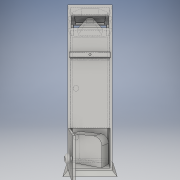
# Autodesk Inventor part: hologram display version 2
Saved by Autodesk Inventor 2016 (Build 200138000, 138)
## iProperties
Created: 2017-10-03
Part Number: hologram display version 2
Material: Generic
Document SubType Name: Modeling
Designer: student
Density: 1 g/cm^3
Appearance: Default
Author: student
Autodesk Inventor part; units mm, degrees
ref_plane "YZ Plane" through (0, 0, 0) normal (1, 0, 0) x (0, 1, 0)
ref_plane "XZ Plane" through (0, 0, 0) normal (0, 1, 0) x (-1, 0, 0)
sketch "Sketch1" plane through (0, 0, 0) normal (0, 0, 1) x (1, 0, 0)
  line L0 (-254, -861.9632) -> (254, -861.9632)
  line L1 (254, -861.9632) -> (254, 763.6368)
  line L2 (254, 763.6368) -> (-254, 763.6368)
  line L3 (-254, 763.6368) -> (-254, -861.9632)
  line L4 (-254, 763.6368) -> (254, 763.6368)
  line L5 (228.6, 763.6368) -> (228.6, -861.9632)
  line L6 (-228.6, 763.6368) -> (-228.6, -861.9632)
  line L7 (-228.6, -836.5632) -> (228.6, -836.5632)
  line L8 (-228.6, 738.2368) -> (228.6, 738.2368)
  line L9 (-254, -861.9632) -> (-304.8, -861.9632)
  line L10 (304.8, -861.9632) -> (304.8, -912.7632)
  line L11 (304.8, -912.7632) -> (-304.8, -912.7632)
  line L12 (-304.8, -912.7632) -> (-304.8, -861.9632)
  line L13 (254, -861.9632) -> (304.8, -861.9632)
  point P0 (0, 0)
  point P1 (0, 0)
  point P2 (0, 738.2368)
  dimension "d0" = 1625.6
  dimension "d1" = 508
  dimension "d3" = 25.4
  dimension "d4" = 25.4
  dimension "d5" = 25.4
  dimension "d6" = 25.4
  dimension "d7" = 50.8
  dimension "d8" = 50.8
  dimension "d19" = 50.8
  constraints: 28 end point, 8 point on line, 5 perpendicular, 4 horizontal, 3 parallel, 1 midpoint, 1 vertical alignment
  measures "d0" distance of L0.end L1.end
  measures "d1" distance of L0.start L0.end
  measures "d3" distance between parallel lines of L1 L5
  measures "d4" distance between parallel lines of L3 L6
  measures "d5" distance between parallel lines of L0 L7
  measures "d6" distance between parallel lines of L8 L2
  measures "d7" distance of L0.start L9.end
  measures "d8" distance of L10.start L10.end
  measures "d19" distance of L0.end L10.start
extrude "Extrusion1" add sketch "Sketch1" along normal blind 406.4 contours L3 L2 L6 L0 | L0 L13 L10 L11 L12 L9 | L6 L7 L5 L0 | L5 L2 L1 L0 | L2 L5 L8 L6
sketch "Sketch2" plane through (0, 0, 406.4) normal (0, 0, 1) x (1, 0, 0)
  line L0 (-304.8, -861.9632) -> (-304.8, -912.7632) projected
  line L1 (-304.8, -912.7632) -> (304.8, -912.7632) projected
  line L2 (-304.8, -861.9632) -> (304.8, -861.9632)
  line L3 (304.8, -861.9632) -> (304.8, -912.7632)
  line L4 (304.8, -912.7632) -> (-304.8, -912.7632)
  line L5 (-304.8, -912.7632) -> (-304.8, -861.9632)
  point P0 (0, 0)
  constraints: 8 end point, 2 parallel, 1 horizontal, 1 perpendicular
extrude "Extrusion2" add sketch "Sketch2" along normal blind 50.8
sketch "Sketch3" plane through (0, 0, 0) normal (0, 0, -1) x (-1, 0, 0)
  line L0 (-304.8, -912.7632) -> (-304.8, -861.9632) projected
  line L1 (304.8, -912.7632) -> (-304.8, -912.7632) projected
  line L2 (-304.8, -861.9632) -> (304.8, -861.9632)
  line L3 (304.8, -861.9632) -> (304.8, -912.7632)
  line L4 (304.8, -912.7632) -> (-304.8, -912.7632)
  line L5 (-304.8, -912.7632) -> (-304.8, -861.9632)
  point P0 (0, 0)
  constraints: 8 end point, 2 parallel, 1 horizontal, 1 perpendicular
extrude "Extrusion3" add sketch "Sketch3" along normal blind 50.8
sketch "Sketch4" plane through (228.6, -836.5632, 0) normal (-1, 0, 0) x (0, 0, 1)
  line L0 (0, 1574.8) -> (406.4, 1574.8) projected
  line L1 (0, 0) -> (25.4, 0)
  line L2 (25.4, 0) -> (25.4, 1574.8)
  line L3 (25.4, 1574.8) -> (0, 1574.8)
  line L4 (0, 1574.8) -> (0, 0)
  point P0 (0, 836.5632)
  dimension "d26" = 25.4
  constraints: 8 end point, 2 parallel, 1 horizontal, 1 perpendicular, 1 point on line
  measures "d26" distance between parallel lines of L4 L2
extrude "Extrusion4" add sketch "Sketch4" along normal blind 457.2
chamfer "Chamfer1" distance 50.8 angle 45 4 edges at (304.8, -861.9632, 203.2) (0, -861.9632, 457.2) (-304.8, -861.9632, 203.2) (0, -861.9632, -50.8)
sketch "Sketch5" plane through (-254, 763.6368, 0) normal (0, 1, 0) x (1, 0, 0)
  line L0 (403.225, -53.975) -> (403.225, -352.425)
  line L1 (403.225, -352.425) -> (104.775, -352.425)
  line L2 (104.775, -352.425) -> (104.775, -53.975)
  line L3 (104.775, -53.975) -> (403.225, -53.975)
  line L4 (508, 0) -> (0, 0) projected
  line L5 (508, 0) -> (508, -406.4) projected
  point P0 (254, 0)
  point P1 (254, -203.2)
  point P2 (254, 0)
  point P3 (508, -203.2)
  dimension "d32" = 298.45
  constraints: 8 end point, 2 midpoint, 1 horizontal alignment, 1 vertical alignment, 9 other
  measures "d32" distance of L0.start L0.end
ref_plane "Work Plane1" through (-254, 928.7368, 0) normal (0, 1, 0) x (1, 0, 0)
sketch "Sketch6" plane through (-254, 928.7368, 0) normal (0, 1, 0) x (1, 0, 0)
  line L0 (285.75, -171.45) -> (285.75, -234.95)
  line L1 (285.75, -234.95) -> (222.25, -234.95)
  line L2 (222.25, -234.95) -> (222.25, -171.45)
  line L3 (222.25, -171.45) -> (285.75, -171.45)
  line L4 (508, 0) -> (0, 0) projected
  line L5 (508, 0) -> (508, -406.4) projected
  point P0 (254, 0)
  point P1 (254, -203.2)
  point P2 (254, 0)
  point P3 (508, -203.2)
  dimension "d34" = 63.5
  constraints: 8 end point, 2 midpoint, 1 horizontal alignment, 1 parallel, 1 vertical alignment, 9 other
  measures "d34" distance of L0.start L0.end
loft "Loft1" add profiles "Sketch6", "Sketch5"
sketch "Sketch7" plane through (-31.75, 928.7368, 171.45) normal (0, 1, 0) x (1, 0, 0)
  line L0 (-173.99, 137.16) -> (237.49, 137.16)
  line L1 (237.49, 137.16) -> (237.49, -200.66)
  line L2 (237.49, -200.66) -> (-173.99, -200.66)
  line L3 (-173.99, -200.66) -> (-173.99, 137.16)
  line L4 (-173.99, 137.16) -> (237.49, -200.66) construction
  line L5 (237.49, 137.16) -> (-173.99, -200.66) construction
  line L6 (285.75, 171.45) -> (285.75, -234.95) projected
  point P0 (31.75, 171.45)
  point P1 (31.75, -31.75)
  point P2 (31.75, 137.16)
  point P3 (31.75, -31.75)
  point P4 (31.75, -31.75)
  point P5 (237.49, -31.75)
  point P6 (285.75, -31.75)
  dimension "d39" = 337.82
  dimension "d40" = 411.48
  constraints: 12 end point, 7 midpoint, 2 horizontal alignment, 2 parallel, 2 vertical alignment, 1 horizontal, 1 perpendicular
  measures "d39" distance of L0.end L1.end
  measures "d40" distance of L0.start L0.end
extrude "Extrusion5" add sketch "Sketch7" along normal blind 65.024
sketch "Sketch8" plane through (-205.74, 928.7368, 372.11) normal (0, 0, 1) x (1, 0, 0)
  line L0 (102.87, 65.024) -> (308.61, 65.024)
  line L1 (308.61, 65.024) -> (411.48, 23.876)
  line L2 (102.87, 65.024) -> (0, 23.876)
  line L3 (0, 23.876) -> (0, 65.024)
  line L4 (411.48, 65.024) -> (0, 65.024) projected
  line L5 (0, 65.024) -> (102.87, 65.024)
  line L6 (308.61, 65.024) -> (411.48, 65.024)
  line L7 (411.48, 65.024) -> (411.48, 23.876)
  point P0 (205.74, -928.7368)
  point P1 (205.74, 65.024)
  point P2 (205.74, 0)
  point P3 (411.48, 0)
  dimension "d49" = 205.74
  dimension "d50" = 23.876
  constraints: 14 end point, 3 perpendicular, 1 horizontal, 1 midpoint, 1 vertical alignment
  measures "d49" distance of L0.start L0.end
  measures "d50" distance of point (411.48, 0) L1.end
extrude "Extrusion6" cut sketch "Sketch8" against normal blind 649.351
sketch "Sketch9" plane through (-254, 763.6368, 0) normal (0, 1, 0) x (1, 0, 0)
  line L0 (508, 0) -> (0, 0) projected
  line L1 (38.1, 0) -> (38.1, -38.1)
  line L2 (38.1, -38.1) -> (0, -38.1)
  line L3 (0, -38.1) -> (0, 0)
  line L4 (0, 0) -> (38.1, 0)
  line L5 (508, 0) -> (508, -406.4) projected
  line L6 (508, 0) -> (508, -38.1)
  line L7 (508, -38.1) -> (469.9, -38.1)
  line L8 (469.9, -38.1) -> (469.9, 0)
  line L9 (469.9, 0) -> (508, 0)
  line L10 (0, 0) -> (0, -406.4) projected
  line L11 (0, -406.4) -> (0, -368.3)
  line L12 (0, -368.3) -> (38.1, -368.3)
  line L13 (38.1, -368.3) -> (38.1, -406.4)
  line L14 (38.1, -406.4) -> (0, -406.4)
  line L15 (508, -406.4) -> (469.9, -406.4)
  line L16 (469.9, -406.4) -> (469.9, -368.3)
  line L17 (469.9, -368.3) -> (508, -368.3)
  line L18 (508, -368.3) -> (508, -406.4)
  point P0 (254, 0)
  point P1 (19.05, -19.05)
  point P2 (19.05, 0)
  point P3 (0, -19.05)
  point P4 (488.95, -19.05)
  point P5 (488.95, 0)
  point P6 (19.05, -387.35)
  point P7 (19.05, -406.4)
  point P8 (488.95, -387.35)
  dimension "d53" = 38.1
  dimension "d54" = 38.1
  dimension "d55" = 38.1
  dimension "d56" = 38.1
  constraints: 32 end point, 4 midpoint, 3 horizontal alignment, 1 point on line, 1 vertical, 1 vertical alignment, 36 other
  measures "d53" distance of L1.start L1.end
  measures "d54" distance of L6.end L7.end
  measures "d55" distance of L12.end L13.end
  measures "d56" distance of L16.end L17.end
extrude "Extrusion7" add sketch "Sketch9" along normal blind 139.7
sketch "Sketch10" plane through (-254, 903.3368, 0) normal (0, 1, 0) x (1, 0, 0)
  line L0 (469.9, -406.4) -> (508, -406.4) projected
  line L1 (0, 0) -> (508, 0)
  line L2 (508, 0) -> (508, -406.4)
  line L3 (508, -406.4) -> (0, -406.4)
  line L4 (0, -406.4) -> (0, 0)
  line L5 (69.85, -31.75) -> (438.15, -31.75)
  line L6 (438.15, -31.75) -> (438.15, -374.65)
  line L7 (438.15, -374.65) -> (69.85, -374.65)
  line L8 (69.85, -374.65) -> (69.85, -31.75)
  line L9 (469.9, -368.3) -> (469.9, -406.4) projected
  line L10 (38.1, -406.4) -> (38.1, -368.3) projected
  line L11 (38.1, -38.1) -> (38.1, 0) projected
  line L12 (469.9, 0) -> (469.9, -38.1) projected
  point P0 (254, 0)
  dimension "d59" = 31.75
  dimension "d60" = 31.75
  dimension "d61" = 31.75
  dimension "d62" = 31.75
  dimension "d63" = 31.75
  dimension "d64" = 31.75
  constraints: 16 end point, 4 parallel, 2 horizontal, 2 perpendicular
  measures "d59" distance from line of L9 L6.end
  measures "d60" distance between parallel lines of L3 L7
  measures "d61" distance between parallel lines of L10 L8
  measures "d62" distance between parallel lines of L11 L8
  measures "d63" distance between parallel lines of L12 L6
  measures "d64" distance between parallel lines of L1 L5
extrude "Extrusion8" add sketch "Sketch10" along normal blind 25.4
sketch "Sketch11" plane through (-228.6, -836.5632, 406.4) normal (1, 0, 0) x (0, 0, -1)
  line L0 (0, 0) -> (0, 1574.8) projected
  line L1 (0, 1574.8) -> (25.4, 1574.8)
  line L2 (25.4, 1574.8) -> (25.4, 457.2)
  line L3 (25.4, 457.2) -> (0, 457.2)
  line L4 (0, 457.2) -> (0, 1574.8)
  line L5 (381, 0) -> (0, 0) projected
  point P0 (406.4, 836.5632)
  dimension "d67" = 25.4
  dimension "d68" = 457.2
  constraints: 8 end point, 2 parallel, 1 horizontal, 1 perpendicular
  measures "d67" distance between parallel lines of L0 L2
  measures "d68" distance between parallel lines of L5 L3
extrude "Extrusion9" add sketch "Sketch11" along normal blind 457.2
sketch "Sketch12" plane through (-254, 928.7368, 0) normal (0, 1, 0) x (1, 0, 0)
  line L0 (0, 0) -> (508, 0)
  line L1 (508, 0) -> (508, -406.4)
  line L2 (508, -406.4) -> (0, -406.4)
  line L3 (0, -406.4) -> (0, 0)
  line L4 (25.4, -25.4) -> (482.6, -25.4)
  line L5 (482.6, -25.4) -> (482.6, -381)
  line L6 (482.6, -381) -> (25.4, -381)
  line L7 (25.4, -381) -> (25.4, -25.4)
  line L8 (304.8, 0) -> (304.8, -25.4)
  line L9 (304.8, -25.4) -> (203.2, -25.4)
  line L10 (203.2, -25.4) -> (203.2, 0)
  point P0 (254, 0)
  dimension "d71" = 25.4
  dimension "d72" = 25.4
  dimension "d73" = 25.4
  dimension "d74" = 25.4
  constraints: 22 end point, 5 parallel, 3 point on line, 2 horizontal, 2 perpendicular
  measures "d71" distance between parallel lines of L0 L4
  measures "d72" distance between parallel lines of L3 L7
  measures "d73" distance between parallel lines of L1 L5
  measures "d74" distance between parallel lines of L2 L6
extrude "Extrusion10" add sketch "Sketch12" along normal blind 71.12 contours L0 L10 L4 L7 L6 L5 L8 L1 L2 L3
sketch "Sketch13" plane through (0, 0, 406.4) normal (0, 0, 1) x (1, 0, 0)
  line L0 (-254, 999.8568) -> (254, 999.8568) projected
  line L1 (-254, 999.8568) -> (254, 999.8568)
  line L2 (254, 999.8568) -> (254, 1025.2568)
  line L3 (254, 1025.2568) -> (-254, 1025.2568)
  line L4 (-254, 1025.2568) -> (-254, 999.8568)
  point P0 (0, 0)
  dimension "d78" = 25.4
  constraints: 8 end point, 2 parallel, 1 horizontal, 1 perpendicular
  measures "d78" distance of L1.end L2.end
extrude "Extrusion11" add sketch "Sketch13" against normal blind 406.4
sketch "Sketch14" plane through (-228.6, -836.5632, 406.4) normal (0, 1, 0) x (1, 0, 0)
  line L0 (3.5018, 227.1968) -> (364.1271, 13.6687)
  line L1 (364.1271, 13.6687) -> (451.4795, 161.1972)
  line L2 (451.4795, 161.1972) -> (90.8542, 374.7253)
  line L3 (90.8542, 374.7253) -> (3.5018, 227.1968)
  point P0 (228.6, 406.4)
  point P1 (234.9388, 199.449)
  dimension "d81" = 171.45
  dimension "d82" = 419.1
  constraints: 8 end point, 2 parallel, 1 perpendicular
  measures "d81" distance of L0.end L1.end
  measures "d82" distance of L0.start L0.end
extrude "Extrusion12" add sketch "Sketch14" along normal blind 355.6
fillet "Fillet1" radius 104.775 1 edges at (179.2033, -480.9632, 318.9671)
sketch "Sketch16" plane through (0, 0, 0) normal (0, 0, -1) x (-1, 0, 0)
  circle A0 centre (182.88, -557.1632) radius 38.1
  line L0 (-254, -861.9632) -> (254, -861.9632) projected
  line L1 (254, -861.9632) -> (254, 1025.2568) projected
  circle A1 centre (182.88, 77.8368) radius 38.1
  point P0 (0, 0)
  dimension "d95" = 304.8
  dimension "d96" = 76.2
  dimension "d99" = 71.12
  dimension "d100" = 939.8
  dimension "d136" = 71.12
  constraints: 2 centre point
  measures "d95" distance from line of L0 A0.centre
  measures "d96" diameter of A0
  measures "d99" distance from line of L1 A0.centre
  measures "d100" distance from line of L0 A1.centre
  measures "d136" distance from line of L1 A1.centre
extrude "Extrusion13" cut sketch "Sketch16" against normal blind 41.275
sketch "Sketch17" plane through (0, 0, 406.4) normal (0, 0, 1) x (1, 0, 0)
  line L0 (-254, 763.6368) -> (-215.9, 763.6368) projected
  line L1 (-228.6, 484.2368) -> (228.6, 484.2368)
  line L2 (228.6, 484.2368) -> (228.6, 420.7368)
  line L3 (228.6, -379.3632) -> (228.6, 738.2368) projected
  line L4 (228.6, 420.7368) -> (-228.6, 420.7368)
  line L5 (-228.6, 420.7368) -> (-228.6, 484.2368)
  line L6 (215.9, 763.6368) -> (-215.9, 763.6368) projected
  point P0 (0, 0)
  point P1 (0, 484.2368)
  point P2 (0, 763.6368)
  dimension "d104" = 63.5
  dimension "d113" = 457.2
  dimension "d114" = 279.4
  constraints: 8 end point, 2 midpoint, 2 perpendicular, 1 collinear, 1 horizontal, 1 vertical alignment
  measures "d104" distance of L4.end L1.start
  measures "d113" distance of L2.end L4.end
  measures "d114" distance between parallel lines of L6 L1
extrude "Extrusion14" cut sketch "Sketch17" against normal blind 98.425
sketch "Sketch18" plane through (0, 0, 406.4) normal (0, 0, 1) x (1, 0, 0)
  line L0 (228.6, 484.2368) -> (228.6, 420.7368) projected
  line L1 (-228.6, 420.7368) -> (228.6, 420.7368)
  line L2 (228.6, 420.7368) -> (228.6, 433.4368)
  line L3 (228.6, 433.4368) -> (-228.6, 433.4368)
  line L4 (-228.6, 433.4368) -> (-228.6, 420.7368)
  point P0 (0, 0)
  dimension "d107" = 12.7
  constraints: 8 end point, 2 parallel, 1 horizontal, 1 perpendicular, 1 point on line
  measures "d107" distance of L3.end L1.start
extrude "Extrusion15" add sketch "Sketch18" against normal blind 266.7 and the other way blind 76.2
sketch "Sketch19" plane through (-228.6, 433.4368, 406.4) normal (0, 1, 0) x (1, 0, 0)
  line L0 (0, 0) -> (0, -76.2) projected
  line L1 (0, 266.7) -> (0, 254)
  line L2 (457.2, 266.7) -> (0, 266.7)
  line L3 (0, 266.7) -> (0, 254)
  line L4 (0, 254) -> (457.2, 254)
  line L5 (457.2, 254) -> (457.2, 266.7)
  point P0 (228.6, 406.4)
  point P1 (0, 25.4)
  point P2 (0, 368.3)
  dimension "d115" = 12.7
  constraints: 10 end point, 2 parallel, 1 horizontal, 1 perpendicular, 1 point on line
  measures "d115" distance of L4.end L2.start
extrude "Extrusion16" add sketch "Sketch19" along normal blind 12.7
sketch "Sketch20" plane through (-228.6, -836.5632, 406.4) normal (0, 1, 0) x (1, 0, 0)
  line L0 (457.2, 0) -> (0, 0) projected
  line L1 (0, 0) -> (89.0436, -448.4452)
  line L2 (89.0436, -448.4452) -> (64.13, -453.392)
  line L3 (64.13, -453.392) -> (-24.9136, -4.9469)
  line L4 (-24.9136, -4.9469) -> (0, 0)
  point P0 (228.6, 406.4)
  dimension "d116" = 457.2
  dimension "d117" = 25.4
  constraints: 8 end point, 2 parallel, 1 perpendicular
  measures "d116" distance of L0.end L1.end
  measures "d117" distance of L1.end L2.end
extrude "Extrusion17" add sketch "Sketch20" along normal blind 457.2
sketch "Sketch21" plane through (-164.47, -836.5632, 859.792) normal (-0.9808512, 0, 0.1947586) x (0.1947586, 0, 0.9808512)
  circle A0 centre (-50.8, 228.6) radius 19.05
  line L0 (0, 0) -> (0, 457.2) projected
  point P0 (-811.2961, 836.5632)
  point P1 (0, 228.6)
  dimension "d120" = 38.1
  dimension "d135" = 50.8
  constraints: 1 centre point, 1 horizontal alignment, 1 midpoint
  measures "d120" diameter of A0
  measures "d135" distance of point (0, 228.6) A0.centre
extrude "Extrusion18" add sketch "Sketch21" along normal blind 19.05
sketch "Sketch22" plane through (-193.0489, -607.9632, 813.6749) normal (-0.9808512, 0, 0.1947586) x (0.1947586, 0, 0.9808512)
  circle A0 centre (0, 0) radius 19.05 projected
  circle A1 centre (0, 0) radius 50.8
  point P0 (-760.4961, 607.9632)
  dimension "d123" = 101.6
  constraints: 1 centre point, 1 coincident
  measures "d123" diameter of A1
extrude "Extrusion19" add sketch "Sketch22" along normal blind 50.8 contours A0 | A1
fillet "Fillet2" radius 25.4 2 edges at (-202.9427, -607.9632, 763.8477) (-252.7699, -607.9632, 773.7414)
sketch "Sketch23" plane through (-228.6, 433.4368, 482.6) normal (0, 1, 0) x (1, 0, 0)
  line L0 (457.2, 76.2) -> (457.2, 0) projected
  line L1 (0, 0) -> (457.2, 0)
  line L2 (457.2, 0) -> (457.2, 12.7)
  line L3 (457.2, 12.7) -> (0, 12.7)
  line L4 (0, 12.7) -> (0, 0)
  point P0 (228.6, 482.6)
  dimension "d129" = 12.7
  constraints: 8 end point, 2 parallel, 1 horizontal, 1 perpendicular, 1 point on line
  measures "d129" distance of L3.end L1.start
extrude "Extrusion20" add sketch "Sketch23" along normal blind 45.72
sketch "Sketch24" plane through (0, 0, 482.6) normal (0, 0, 1) x (1, 0, 0)
  circle A0 centre (0, 449.9468) radius 12.7
  line L0 (228.6, 420.7368) -> (228.6, 479.1568) projected
  point P0 (0, 0)
  point P1 (228.6, 449.9468)
  point P2 (228.6, 449.9468)
  dimension "d132" = 25.4
  constraints: 2 horizontal alignment, 2 midpoint, 1 centre point
  measures "d132" diameter of A0
extrude "Extrusion21" cut sketch "Sketch24" against normal blind 33.3375
body "Solid1"
